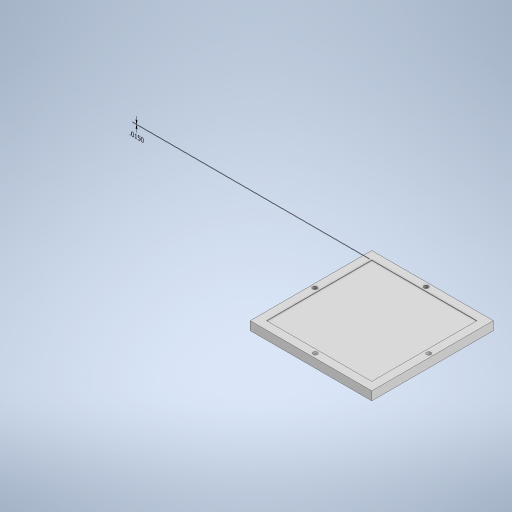
# Autodesk Inventor part: bottom plate
Saved by Autodesk Inventor 2024.2 (Build 282272000, 272)
## iProperties
Created: 2024-11-01
Part Number: bottom plate
Material: Generic
Document SubType Name: Modeling
Designer: Tom
Density: 1 g/cm^3
Appearance: Default
Author: Tom
Autodesk Inventor part; units mm, degrees
ref_plane "YZ Plane" through (0, 0, 0) normal (1, 0, 0) x (0, 1, 0)
ref_plane "XZ Plane" through (0, 0, 0) normal (0, 1, 0) x (-1, 0, 0)
ref_plane "XY Plane" through (0, 0, 0) normal (0, 0, 1) x (1, 0, 0)
sketch "Sketch1" plane through (0, 0, 0) normal (0, 1, 0) x (-1, 0, 0)
  line L0 (0, 0) -> (88.9, 0)
  line L1 (88.9, 0) -> (88.9, -88.9)
  line L2 (88.9, -88.9) -> (0, -88.9)
  line L3 (0, -88.9) -> (0, 0)
  dimension "d0" = 88.9
  dimension "d1" = 88.9
  constraints: 8 end point, 2 parallel, 1 horizontal, 1 perpendicular
  measures "d0" distance of L0.end L1.end
  measures "d1" distance of L1.end L2.end
extrude "Extrusion1" add sketch "Sketch1" along normal blind 6.35
shell "Shell1" thickness 5.969 removed faces 1 at (-29.6333, 6.35, -29.6333)
sketch "Sketch2" plane through (0, 6.35, 0) normal (0, 1, 0) x (1, 0, 0)
  circle A0 centre (-44.45, 3.1115) radius 1.5875
  line L0 (-88.9, 88.9) -> (-88.9, 0) projected
  line L1 (-5.969, 5.969) -> (-82.931, 5.969) projected
  circle A1 centre (-86.0425, 44.45) radius 1.5875
  line L2 (-88.9, 0) -> (0, 0) projected
  circle A2 centre (-2.8575, 44.45) radius 1.5875
  line L3 (0, 0) -> (0, 88.9) projected
  circle A3 centre (-46.0375, 85.7885) radius 1.5875
  line L4 (-82.931, 82.931) -> (-5.969, 82.931) projected
  dimension "d8" = 3.175
  dimension "d10" = 2.8575
  dimension "d11" = 3.175
  dimension "d12" = 2.8575
  dimension "d13" = 44.45
  dimension "d14" = 3.175
  dimension "d15" = 2.8575
  dimension "d16" = 3.175
  dimension "d17" = 2.8575
  constraints: 4 centre point
  measures "d8" diameter of A0
  measures "d10" distance from line of L1 A0.centre
  measures "d11" diameter of A1
  measures "d12" distance from line of L0 A1.centre
  measures "d13" distance from line of L2 A1.centre
  measures "d14" diameter of A2
  measures "d15" distance from line of L3 A2.centre
  measures "d16" diameter of A3
  measures "d17" distance from line of L4 A3.centre
extrude "Extrusion2" cut sketch "Sketch2" against normal blind 3.175
body "Solid1"
